Support Suspension  OUT (Autodesk Fusion 360 design; units mm, degrees)
Autodesk Fusion 360 part; units mm, degrees
note: some values were not read from the file. Chosen so that the rebuilt part matches the saved one: the layout of a text.
sketch "Sketch1" plane through (0, 0, 0) normal (0, 0, 1) x (1, 0, 0)
  line L0 (19.5, 61) -> (-19.5, 61)
  line L1 (-19.5, 61) -> (-19.5, -61)
  line L2 (-19.5, -61) -> (19.5, -61)
  line L3 (19.5, -61) -> (19.5, 61)
  line L4 (19.5, 61) -> (-19.5, -61) construction
  line L5 (-19.5, 61) -> (19.5, -61) construction
  line L6 (-26.5, 61) -> (39.5, 61)
  line L7 (39.5, 61) -> (39.5, 54)
  line L8 (39.5, 54) -> (-26.5, 54)
  line L9 (-26.5, 54) -> (-26.5, 61)
  line L10 (-19.5, 0) -> (19.5, 0) construction
  line L11 (39.5, -54) -> (-26.5, -54)
  line L12 (-26.5, -54) -> (-26.5, -61)
  line L13 (-26.5, -61) -> (39.5, -61)
  line L14 (39.5, -61) -> (39.5, -54)
  line L15 (-19.5, -3.3) -> (19.5, -3.3) construction
  line L16 (0, 0) -> (0, -64.5802) construction
  circle A0 centre (0, -3.3) radius 22.5 construction
  circle A1 centre (0, 19.2) radius 2.1
  circle A2 centre (-19.4856, 7.95) radius 2.1
  circle A3 centre (-19.4856, -14.55) radius 2.1
  circle A4 centre (0, -25.8) radius 2.1
  circle A5 centre (19.4856, -14.55) radius 2.1
  circle A6 centre (19.4856, 7.95) radius 2.1
  circle A7 centre (-19.4856, 7.95) radius 4
  circle A8 centre (-19.4856, -14.55) radius 4
  circle A9 centre (19.4856, 7.95) radius 4
  circle A10 centre (19.4856, -14.55) radius 4
  line L17 (19.4856, 6.7) -> (29.4856, 6.7)
  line L18 (29.4856, 6.7) -> (29.4856, 9.2)
  line L19 (29.4856, 9.2) -> (19.4856, 9.2)
  line L20 (19.4856, 9.2) -> (19.4856, 6.7)
  line L21 (0, 0) -> (0, 19.2) construction
  line L22 (29.4856, 9.2) -> (19.4856, 9.2)
  line L23 (19.4856, 9.2) -> (19.4856, 6.7)
  line L24 (19.4856, 6.7) -> (29.4856, 6.7)
  line L25 (29.4856, 6.7) -> (29.4856, 9.2)
  line L26 (29.4856, 9.2) -> (19.4856, 9.2)
  line L27 (19.4856, 9.2) -> (19.4856, 6.7)
  line L28 (19.4856, 6.7) -> (29.4856, 6.7)
  line L29 (29.4856, 6.7) -> (29.4856, 9.2)
  line L30 (29.4856, -13.3) -> (19.4856, -13.3)
  line L31 (19.4856, -13.3) -> (19.4856, -15.8)
  line L32 (19.4856, -15.8) -> (29.4856, -15.8)
  line L33 (29.4856, -15.8) -> (29.4856, -13.3)
  line L34 (-19.4856, 9.2) -> (-29.4856, 9.2)
  line L35 (-29.4856, 9.2) -> (-29.4856, 6.7)
  line L36 (-29.4856, 6.7) -> (-19.4856, 6.7)
  line L37 (-19.4856, 6.7) -> (-19.4856, 9.2)
  line L38 (-19.4856, -13.3) -> (-29.4856, -13.3)
  line L39 (-29.4856, -13.3) -> (-29.4856, -15.8)
  line L40 (-29.4856, -15.8) -> (-19.4856, -15.8)
  line L41 (-19.4856, -15.8) -> (-19.4856, -13.3)
  circle A11 centre (0, -3.3) radius 4
  circle A12 centre (0, 51) radius 2.1
  line L42 (0, 61) -> (0, -61) construction
  circle A13 centre (0, -51) radius 2.1
  dimension "d1" = 122
  dimension "d9" = 39
  dimension "d10" = 7
  dimension "d11" = 7
  dimension "d12" = 20
  dimension "d13" = 3.3
  dimension "d14" = 45
  dimension "d15" = 4.2
  dimension "d17" = 360
  dimension "d18" = 8
  dimension "d19" = 8
  dimension "d20" = 8
  dimension "d21" = 8
  dimension "d28" = 2.5
  dimension "d29" = 10
  dimension "d30" = 2.5
  dimension "d31" = 10
  dimension "d32" = 2.5
  dimension "d33" = 10
  dimension "d34" = 2.5
  dimension "d35" = 10
  dimension "d36" = 2.5
  dimension "d37" = 10
  dimension "d38" = 2.5
  dimension "d39" = 10
  dimension "d41" = 8
  dimension "d51" = 4.2
  dimension "d52" = 10
  dimension "d53" = 4.2
  dimension "d54" = 10
  constraint perpendicular L0 L1
  constraint parallel L0 L2
  constraint parallel L1 L3
  constraint horizontal L0
  constraint horizontal L6
  constraint vertical L7
  constraint horizontal L8
  constraint vertical L9
  constraint coincident L0.end L6
  constraint midpoint L1 L10.start
  constraint midpoint L3 L10.end
  constraint symmetric L6.start L10 L12.end
  constraint symmetric L6.end L10 L13.end
  constraint symmetric L7.end L10 L11.start
  constraint symmetric L8.end L10 L11.end
  constraint coincident L1 L15.start
  constraint coincident L3 L15.end
  constraint perpendicular L3 L15
  constraint coincident L16.start L21.start
  constraint perpendicular L11 L16
  constraint midpoint L15 A0.centre
  constraint coincident A0 A1.centre
  constraint concentric A2 A7
  constraint concentric A3 A8
  constraint concentric A6 A9
  constraint concentric A5 A10
  constraint horizontal L17
  constraint vertical L18
  constraint horizontal L19
  constraint vertical L20
  constraint midpoint A6.centre L20
  constraint coincident A1.centre L21.end
  constraint vertical L21
  constraint coincident L16.start L10
  constraint midpoint L16.start L10
  constraint horizontal L24
  constraint vertical L25
  constraint horizontal L22
  constraint vertical L23
  constraint horizontal L28
  constraint vertical L29
  constraint horizontal L26
  constraint vertical L27
  constraint horizontal L32
  constraint vertical L33
  constraint horizontal L30
  constraint vertical L31
  constraint midpoint A5.centre L31
  constraint horizontal L36
  constraint vertical L37
  constraint horizontal L34
  constraint vertical L35
  constraint midpoint A2.centre L37
  constraint horizontal L40
  constraint vertical L41
  constraint horizontal L38
  constraint vertical L39
  constraint midpoint A3.centre L41
  constraint concentric A0 A11
  constraint midpoint L0 L42.start
  constraint midpoint L2 L42.end
  constraint coincident A12.centre L42
  constraint coincident L16 A13.centre
  measures "d1" distance of L0.end L1.end
  measures "d9" distance of L0.start L0.end
  measures "d10" distance of L6.start L8.end
  measures "d11" distance of L0.end L6.start
  measures "d12" distance of L0.start L6.end
  measures "d13" distance of L10 L15
  measures "d14" diameter of A0
  measures "d15" diameter of A1
  measures "d18" diameter of A7
  measures "d19" diameter of A8
  measures "d20" diameter of A9
  measures "d21" diameter of A10
  measures "d28" distance of L17.end L18.end
  measures "d29" distance of L18.end L19.end
  measures "d30" distance of L17.end L18.end
  measures "d31" distance of L19.end L18.end
  measures "d32" distance of L17.end L18.end
  measures "d33" distance of L19.end L18.end
  measures "d34" distance of L32.end L30.start
  measures "d35" distance of L30.end L30.start
  measures "d36" distance of L36.end L34.start
  measures "d37" distance of L34.end L34.start
  measures "d38" distance of L40.end L38.start
  measures "d39" distance of L38.end L38.start
  measures "d41" diameter of A11
  measures "d51" diameter of A12
  measures "d52" distance of L6 A12.centre
  measures "d53" diameter of A13
  measures "d54" distance of L13 A13.centre
extrude "Extrude1" add sketch "Sketch1" along normal blind 7 contours L0 L1 L3 L6 L8 | L3 L6 L7 L8 | L1 L6 L8 L9 | L1 L3 L8 L11 A7 A8 A9 A10 | L3 A6 A9 L19 L22 L26 | L3 A6 A9 | L1 A2 A7 | L1 A2 A7 L34 | A9 L17 L18 L19 L22 L24 L25 L26 L28 L29 | A6 A9 L17 L19 L22 L24 L26 L28 | L3 A6 A9 L17 L24 L28 | A2 A7 L34 L36 | A7 L34 L35 L36 | L3 A5 A10 L30 | L3 A5 A10 | L1 A2 A7 L36 | A10 L30 L32 L33 | A5 A10 L30 L32 | L3 A5 A10 L32 | L1 A3 A8 | L1 A3 A8 L38 | L3 L11 L13 L14 | L1 L2 L3 L11 L13 | A3 A8 L38 L40 | A8 L38 L39 L40 | L1 L11 L12 L13 | L1 A3 A8 L40 makes body 1
chamfer "Chamfer1" distance 11 distance2 6 2 edges at (39.5, -57.5, 7) (39.5, 57.5, 7) measured on face at (-13.5784, 28.7776, 7) measured on face at (-13.5784, 28.7776, 7) on bodies 1
chamfer "Chamfer2" distance 6 angle 45 4 edges at (-29.4856, 7.95, 7) (-29.4856, -14.55, 7) (29.4856, 7.95, 7) (29.4856, -14.55, 7) on bodies 1
mirror "Mirror1" about plane through (0, 0, 0) normal (0, 0, 1) of bodies 1 makes body 2
sketch "Sketch3" plane through (0, 0, 7) normal (0, 0, 1) x (-1, 0, 0)
  line L0 (-23.4856, 15.8) -> (-23.4856, 13.3)
  line L1 (-23.4856, 13.3) -> (-23.2852, 13.3)
  arc A0 (-23.2852, 13.3) -> (-19.5, 10.55) centre (-19.4856, 14.55) ccw
  line L2 (-19.5, 10.55) -> (-19.5, -3.95)
  arc A1 (-19.5, -3.95) -> (-23.2852, -6.7) centre (-19.4856, -7.95) ccw
  line L3 (-23.2852, -6.7) -> (-23.4856, -6.7)
  line L4 (-23.4856, -6.7) -> (-23.4856, -9.2)
  line L5 (-23.4856, -9.2) -> (-23.2852, -9.2)
  arc A2 (-23.2852, -9.2) -> (-19.5, -11.95) centre (-19.4856, -7.95) ccw
  line L6 (-19.5, -11.95) -> (-19.5, -54)
  line L7 (-19.5, -54) -> (-28.5, -54)
  line L8 (-28.5, -54) -> (-28.5, -61)
  line L9 (-28.5, -61) -> (26.5, -61)
  line L10 (26.5, -61) -> (26.5, -54)
  line L11 (26.5, -54) -> (19.5, -54)
  line L12 (19.5, -54) -> (19.5, -11.95)
  arc A3 (19.5, -11.95) -> (23.2852, -9.2) centre (19.4856, -7.95) ccw
  line L13 (23.2852, -9.2) -> (23.4856, -9.2)
  line L14 (23.4856, -9.2) -> (23.4856, -6.7)
  line L15 (23.4856, -6.7) -> (23.2852, -6.7)
  arc A4 (23.2852, -6.7) -> (19.5, -3.95) centre (19.4856, -7.95) ccw
  line L16 (19.5, -3.95) -> (19.5, 10.55)
  arc A5 (19.5, 10.55) -> (23.2852, 13.3) centre (19.4856, 14.55) ccw
  line L17 (23.2852, 13.3) -> (23.4856, 13.3)
  line L18 (23.4856, 13.3) -> (23.4856, 15.8)
  line L19 (23.4856, 15.8) -> (23.2852, 15.8)
  arc A6 (23.2852, 15.8) -> (19.5, 18.55) centre (19.4856, 14.55) ccw
  line L20 (19.5, 18.55) -> (19.5, 54)
  line L21 (19.5, 54) -> (26.5, 54)
  line L22 (26.5, 54) -> (26.5, 61)
  line L23 (26.5, 61) -> (-28.5, 61)
  line L24 (-28.5, 61) -> (-28.5, 54)
  line L25 (-28.5, 54) -> (-19.5, 54)
  line L26 (-19.5, 54) -> (-19.5, 18.55)
  arc A7 (-19.5, 18.55) -> (-23.2852, 15.8) centre (-19.4856, 14.55) ccw
  line L27 (-23.2852, 15.8) -> (-23.4856, 15.8)
  circle A8 centre (0, -19.2) radius 2.1
  circle A9 centre (0, 25.8) radius 2.1
  circle A10 centre (0, 3.3) radius 4
  circle A11 centre (-19.4856, 14.55) radius 2.1
  circle A12 centre (-19.4856, -7.95) radius 2.1
  circle A13 centre (19.4856, -7.95) radius 2.1
  circle A14 centre (19.4856, 14.55) radius 2.1
  line L28 (11.6283, 20.1017) -> (-10.8571, 20.1017) construction
  line L29 (-10.8571, 20.1017) -> (-10.8571, 10.1017) construction
  line L30 (-10.8571, 10.1017) -> (11.6283, 10.1017) construction
  line L31 (11.6283, 10.1017) -> (11.6283, 20.1017) construction
  line L32 (6.0122, -4.7799) -> (-5.5845, -4.7799) construction
  line L33 (-5.5845, -4.7799) -> (-5.5845, -14.7799) construction
  line L34 (-5.5845, -14.7799) -> (6.0122, -14.7799) construction
  line L35 (6.0122, -14.7799) -> (6.0122, -4.7799) construction
  circle A15 centre (0, 51) radius 2.1
  circle A16 centre (0, -51) radius 2.1
  text T0 "Right" font "Arial" height 10 align ink ink in box 0 x 0 at (11.6183, 20.0817) x (-1, 0) y (0, -1) spacing 1 height is em
  text T1 "Up" font "Arial" height 10 align ink ink in box 0 x 0 at (6.0022, -4.7999) x (-1, 0) y (0, -1) spacing 1 height is em
  constraint perpendicular L28 L29
  constraint parallel L28 L30
  constraint parallel L29 L31
  constraint perpendicular L32 L33
  constraint parallel L32 L34
  constraint parallel L33 L35
extrude "Extrude3" cut sketch "Sketch3" against normal blind 1 text T0 T1 bodies 1
sketch "Sketch4" plane through (0, 0, -7) normal (0, 0, -1) x (1, 0, 0)
  circle A0 centre (-19.4856, 14.55) radius 2.1
  circle A1 centre (-19.4856, -7.95) radius 2.1
  circle A2 centre (19.4856, -7.95) radius 2.1
  circle A3 centre (19.4856, 14.55) radius 2.1
  circle A4 centre (0, 3.3) radius 4
  circle A5 centre (0, 25.8) radius 2.1
  circle A6 centre (0, -19.2) radius 2.1
  line L0 (23.4856, 13.3) -> (23.4856, 15.8)
  line L1 (23.4856, 15.8) -> (23.2852, 15.8)
  arc A7 (23.2852, 15.8) -> (19.5, 18.55) centre (19.4856, 14.55) ccw
  line L2 (19.5, 18.55) -> (19.5, 54)
  line L3 (19.5, 54) -> (28.5, 54)
  line L4 (28.5, 54) -> (28.5, 61)
  line L5 (28.5, 61) -> (-26.5, 61)
  line L6 (-26.5, 61) -> (-26.5, 54)
  line L7 (-26.5, 54) -> (-19.5, 54)
  line L8 (-19.5, 54) -> (-19.5, 18.55)
  arc A8 (-19.5, 18.55) -> (-23.2852, 15.8) centre (-19.4856, 14.55) ccw
  line L9 (-23.2852, 15.8) -> (-23.4856, 15.8)
  line L10 (-23.4856, 15.8) -> (-23.4856, 13.3)
  line L11 (-23.4856, 13.3) -> (-23.2852, 13.3)
  arc A9 (-23.2852, 13.3) -> (-19.5, 10.55) centre (-19.4856, 14.55) ccw
  line L12 (-19.5, 10.55) -> (-19.5, -3.95)
  arc A10 (-19.5, -3.95) -> (-23.2852, -6.7) centre (-19.4856, -7.95) ccw
  line L13 (-23.2852, -6.7) -> (-23.4856, -6.7)
  line L14 (-23.4856, -6.7) -> (-23.4856, -9.2)
  line L15 (-23.4856, -9.2) -> (-23.2852, -9.2)
  arc A11 (-23.2852, -9.2) -> (-19.5, -11.95) centre (-19.4856, -7.95) ccw
  line L16 (-19.5, -11.95) -> (-19.5, -54)
  line L17 (-19.5, -54) -> (-26.5, -54)
  line L18 (-26.5, -54) -> (-26.5, -61)
  line L19 (-26.5, -61) -> (28.5, -61)
  line L20 (28.5, -61) -> (28.5, -54)
  line L21 (28.5, -54) -> (19.5, -54)
  line L22 (19.5, -54) -> (19.5, -11.95)
  arc A12 (19.5, -11.95) -> (23.2852, -9.2) centre (19.4856, -7.95) ccw
  line L23 (23.2852, -9.2) -> (23.4856, -9.2)
  line L24 (23.4856, -9.2) -> (23.4856, -6.7)
  line L25 (23.4856, -6.7) -> (23.2852, -6.7)
  arc A13 (23.2852, -6.7) -> (19.5, -3.95) centre (19.4856, -7.95) ccw
  line L26 (19.5, -3.95) -> (19.5, 10.55)
  arc A14 (19.5, 10.55) -> (23.2852, 13.3) centre (19.4856, 14.55) ccw
  line L27 (23.2852, 13.3) -> (23.4856, 13.3)
  line L28 (6.1305, -3.1229) -> (-5.4662, -3.1229) construction
  line L29 (-5.4662, -3.1229) -> (-5.4662, -13.1229) construction
  line L30 (-5.4662, -13.1229) -> (6.1305, -13.1229) construction
  line L31 (6.1305, -13.1229) -> (6.1305, -3.1229) construction
  line L32 (8.3078, 18.4645) -> (-7.5662, 18.4645) construction
  line L33 (-7.5662, 18.4645) -> (-7.5662, 8.4645) construction
  line L34 (-7.5662, 8.4645) -> (8.3078, 8.4645) construction
  line L35 (8.3078, 8.4645) -> (8.3078, 18.4645) construction
  circle A15 centre (0, 51) radius 2.1
  circle A16 centre (0, -51) radius 2.1
  text T0 "Up" font "Arial" height 10 align ink ink in box 0 x 0 at (6.1205, -3.1429) x (-1, 0) y (0, -1) spacing 1 height is em
  text T1 "Left" font "Arial" height 10 align ink ink in box 0 x 0 at (8.2978, 18.4445) x (-1, 0) y (0, -1) spacing 1 height is em
  constraint perpendicular L28 L29
  constraint parallel L28 L30
  constraint parallel L29 L31
  constraint perpendicular L32 L33
  constraint parallel L32 L34
  constraint parallel L33 L35
extrude "Extrude5" cut sketch "Sketch4" against normal blind 1 text T0 T1 bodies 2
move_body "Move1" bodies 2 to x (1, 0, 0) y (0, 1, 0) z (0, 0, 1) at (0, 0, -30)
copy_body "Body->Comp1" bodies 1 removing the originals makes body 3 in component "Right"
copy_body "Body->Comp2" bodies 2 removing the originals makes body 4 in component "Left"
component "Right" placed x (1, 0, 0) y (0, 1, 0) z (0, 0, 1) at (0, 0, 0)
component "Left" placed x (1, 0, 0) y (0, 1, 0) z (0, 0, 1) at (0, 0, 0)
named bodies: "Right", "Left"
